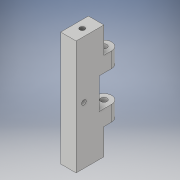
# Autodesk Inventor part: ABI_Führungsblock
Saved by Autodesk Inventor 2018 (Build 220112000, 112)
## iProperties
Created: 2019-11-22
Part Number: ABI_Führungsblock
Material: Generisch
Document SubType Name: Modeling
Designer: maascl
Density: 1 g/cm^3
Appearance: Vorgabe
Author: maascl
Autodesk Inventor part; units mm, degrees
ref_plane "YZ Plane" through (0, 0, 0) normal (1, 0, 0) x (0, 1, 0)
ref_plane "XZ Plane" through (0, 0, 0) normal (0, 1, 0) x (-1, 0, 0)
ref_plane "XY Plane" through (0, 0, 0) normal (0, 0, 1) x (1, 0, 0)
sketch "Skizze1" plane through (0, 0, 0) normal (0, 0, 1) x (1, 0, 0)
  line L0 (5, 14) -> (-5, 14)
  line L1 (-5, 14) -> (-5, -14)
  line L2 (-5, -14) -> (5, -14)
  line L3 (5, -14) -> (5, 14)
  line L4 (5, 14) -> (-5, -14) construction
  line L5 (-5, 14) -> (5, -14) construction
  point P0 (0, 0)
  dimension "d0" = 28
  dimension "d1" = 10
  constraints: 12 end point, 2 midpoint, 2 parallel, 1 horizontal, 1 perpendicular
  measures "d0" distance between parallel lines of L2 L0
  measures "d1" distance between parallel lines of L1 L3
extrude "Extrusion1" add sketch "Skizze1" along normal blind 74
sketch "Skizze2" plane through (-5, -14, 0) normal (-1, 0, 0) x (0, 0, 1)
  line L0 (0, 28) -> (74, 28) projected
  line L1 (0, 28) -> (17, 28)
  line L2 (17, 28) -> (17, 18)
  line L3 (17, 18) -> (0, 18)
  line L4 (0, 18) -> (0, 28)
  line L5 (74, 28) -> (57, 28)
  line L6 (57, 28) -> (57, 18)
  line L7 (57, 18) -> (74, 18)
  line L8 (74, 18) -> (74, 28)
  line L9 (27, 28) -> (47, 28)
  line L10 (47, 28) -> (47, 15)
  line L11 (47, 15) -> (27, 15)
  line L12 (27, 15) -> (27, 28)
  line L13 (0, 0) -> (74, 0) projected
  point P0 (0, 14)
  dimension "d4" = 15
  dimension "d5" = 20
  dimension "d6" = 40
  dimension "d7" = 10
  dimension "d8" = 18
  dimension "d9" = 18
  constraints: 24 end point, 6 parallel, 3 horizontal, 3 perpendicular, 1 point on line
  measures "d4" distance between parallel lines of L13 L11
  measures "d5" distance between parallel lines of L12 L10
  measures "d6" distance between parallel lines of L2 L6
  measures "d7" distance between parallel lines of L12 L2
  measures "d8" distance between parallel lines of L13 L3
  measures "d9" distance between parallel lines of L13 L7
extrude "Extrusion2" cut sketch "Skizze2" against normal blind 74
sketch "Skizze3" plane through (-5, 4, 57) normal (0, 0, 1) x (1, 0, 0)
  line L0 (10, 10) -> (10, 0) projected
  line L1 (10, 0) -> (0, 0) projected
  point P0 (5, -4)
  point P1 (5, 5)
  dimension "d12" = 5
  dimension "d13" = 5
  measures "d12" distance from line of L0 point (5, 5)
  measures "d13" distance from line of L1 point (5, 5)
hole "Bohrung1" at (0, 9, 57) direction (0, 0, -1) diameter 4 end through all
fillet "Rundung1" radius 5 4 edges at (-5, 14, 22) (-5, 14, 52) (5, 14, 52) (5, 14, 22)
sketch "Skizze5" plane through (0, 0, 74) normal (0, 0, 1) x (1, 0, 0)
  line L0 (-5, -14) -> (5, -14) projected
  line L1 (-5, 4) -> (-5, -14) projected
  point P0 (0, 0)
  point P1 (0, -5)
  dimension "d33" = 9
  dimension "d34" = 5
  measures "d33" distance from line of L0 point (0, -5)
  measures "d34" distance from line of L1 point (0, -5)
hole "Bohrung3" at (0, -5, 74) direction (0, 0, -1) diameter 3.242 depth 14 tip angle 118 thread size "M4x0.7" class "6H" standard "ISO Metric profile"
sketch "Skizze6" plane through (0, 0, 0) normal (0, 0, -1) x (-1, 0, 0)
  line L0 (5, 4) -> (5, -14) projected
  line L1 (5, -14) -> (-5, -14) projected
  point P0 (0, 0)
  point P1 (0, -5)
  dimension "d42" = 5
  dimension "d43" = 9
  measures "d42" distance from line of L0 point (0, -5)
  measures "d43" distance from line of L1 point (0, -5)
hole "Bohrung4" at (0, -5, 0) direction (0, 0, 1) diameter 3.242 depth 14 tip angle 118 thread size "M4x0.7" class "6H" standard "ISO Metric profile"
sketch "Skizze7" plane through (5, -14, 74) normal (1, 0, 0) x (0, 0, -1)
  line L0 (74, 0) -> (0, 0) projected
  line L1 (0, 0) -> (0, 18) projected
  point P0 (74, 14)
  point P1 (37, 5)
  dimension "d51" = 5
  dimension "d52" = 37
  measures "d51" distance from line of L0 point (37, 5)
  measures "d52" distance from line of L1 point (37, 5)
hole "Bohrung5" at (5, -9, 37) direction (-1, 0, 0) diameter 3 end through all
